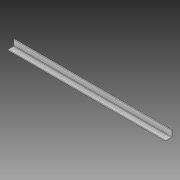
# Autodesk Inventor part: FE-110-001 Floor L Section
Saved by Autodesk Inventor 2021 (Build 250183000, 183)
## iProperties
Created: 2021-01-11
Part Number: FE-110-001 Floor L Section
Material: Aluminum 6061
Document SubType Name: Modeling
Density: 2.7 g/cm^3
Appearance: Aluminum - Dark
Autodesk Inventor part; units mm, degrees
ref_plane "YZ Plane" through (0, 0, 0) normal (1, 0, 0) x (0, 1, 0)
ref_plane "XZ Plane" through (0, 0, 0) normal (0, 1, 0) x (-1, 0, 0)
ref_plane "XY Plane" through (0, 0, 0) normal (0, 0, 1) x (1, 0, 0)
sketch "Sketch1" plane through (0, 0, 0) normal (1, 0, 0) x (0, 1, 0)
  line L0 (0, 0) -> (76.2, 0)
  line L1 (0, 0) -> (0, 76.2)
  arc A0 (6.35, 71.12) -> (1.27, 76.2) centre (1.27, 71.12) ccw
  arc A1 (76.2, 1.27) -> (71.12, 6.35) centre (71.12, 1.27) ccw
  line L2 (76.2, 0) -> (76.2, 1.27)
  line L3 (1.27, 76.2) -> (0, 76.2)
  arc A2 (6.35, 11.43) -> (11.43, 6.35) centre (11.43, 11.43) ccw
  line L4 (6.35, 71.12) -> (6.35, 11.43)
  line L5 (11.43, 6.35) -> (71.12, 6.35)
  dimension "d0" = 76.2
  dimension "d1" = 76.2
  dimension "d2" = 10.16
  dimension "d3" = 10.16
  dimension "d4" = 10.16
  dimension "d5" = 6.35
  constraints: 12 end point, 6 perpendicular, 6 point on circle, 5 tangent, 3 centre point, 1 horizontal, 1 vertical
  measures "d0" distance of L0.start L0.end
  measures "d1" distance of L0.start L1.end
  measures "d2" diameter of A0
  measures "d3" diameter of A1
  measures "d4" diameter of A2
  measures "d5" distance between parallel lines of L1 L4
extrude "Extrusion1" add sketch "Sketch1" along normal mid plane 1828.8
body "Solid1"
